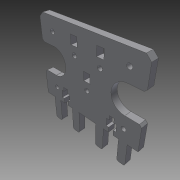
# Autodesk Inventor part: x_carryage_extruder_mount
Saved by Autodesk Inventor 2014 (Build 180170000, 170)
## iProperties
Created: 2014-03-26
Part Number: x_carryage_extruder_mount
Material: Generic
Document SubType Name: Modeling
Designer: buben
Density: 1 g/cm^3
Appearance: Default
Mass: 39.8284 g
Surface Area: 154.479 cm^2
Volume: 39.8284 cm^3
Author: buben
Autodesk Inventor part; units mm, degrees
ref_plane "YZ Plane" through (0, 0, 0) normal (1, 0, 0) x (0, 1, 0)
ref_plane "XZ Plane" through (0, 0, 0) normal (0, 1, 0) x (-1, 0, 0)
ref_plane "XY Plane" through (0, 0, 0) normal (0, 0, 1) x (1, 0, 0)
sketch "Sketch1" plane through (0, 0, 0) normal (0, 1, 0) x (-1, 0, 0)
  line L0 (0, 0) -> (-100, 0)
  line L1 (-100, 0) -> (-100, -24.25)
  line L2 (-100, -24.25) -> (-86, -24.25)
  arc A0 (-86, -50.25) -> (-86, -24.25) centre (-86, -37.25) ccw
  line L3 (-86, -50.25) -> (-100, -50.25)
  line L4 (-100, -50.25) -> (-100, -74.5)
  line L5 (-100, -74.5) -> (0, -74.5)
  line L6 (0, -74.5) -> (0, -50.25)
  line L7 (0, -50.25) -> (-14, -50.25)
  arc A1 (-14, -24.25) -> (-14, -50.25) centre (-14, -37.25) ccw
  line L8 (-14, -24.25) -> (0, -24.25)
  line L9 (0, -24.25) -> (0, 0)
  circle A2 centre (-14, -62.25) radius 2.25
  circle A3 centre (-14, -12.25) radius 2.25
  circle A4 centre (-86, -62.25) radius 2.25
  circle A5 centre (-86, -12.25) radius 2.25
  dimension "d0" = 13
  dimension "d1" = 50
  dimension "d2" = 4.5
  dimension "d3" = 25
  dimension "d5" = 12.25
  dimension "d6" = 100
  dimension "d10" = 14
  constraints: 20 end point, 7 collinear, 6 centre point, 4 parallel, 4 perpendicular, 4 point on circle, 4 tangent, 4 vertical alignment, 3 equal radius, 2 horizontal alignment, 1 horizontal
  measures "d0" radius of A1
  measures "d1" distance of A3.centre A2.centre
  measures "d2" diameter of A2
  measures "d3" distance of A1.centre A2.centre
  measures "d5" distance from line of L5 A2.centre
  measures "d6" distance of L0.start L0.end
  measures "d10" distance from line of L9 A3.centre
extrude "Extrusion1" add sketch "Sketch1" along normal blind 6.5
sketch "Sketch3" plane through (0, 6.5, 0) normal (0, 1, 0) x (1, 0, 0)
  line L0 (100, 74.5) -> (0, 74.5) projected
  line L1 (22.75, 74.5) -> (27.25, 74.5)
  line L2 (27.25, 58.2) -> (22.75, 58.2)
  line L3 (29.75, 69.5) -> (29.75, 62.2)
  line L4 (20.25, 62.2) -> (20.25, 69.5)
  line L5 (27.25, 74.5) -> (27.25, 69.5)
  line L6 (27.25, 62.2) -> (27.25, 58.2)
  line L7 (22.75, 58.2) -> (22.75, 62.2)
  line L8 (22.75, 69.5) -> (22.75, 74.5)
  line L9 (20.25, 69.5) -> (22.75, 69.5)
  line L10 (27.25, 69.5) -> (29.75, 69.5)
  line L11 (29.75, 62.2) -> (27.25, 62.2)
  line L12 (22.75, 62.2) -> (20.25, 62.2)
  line L13 (72.75, 74.5) -> (77.25, 74.5)
  line L14 (77.25, 58.2) -> (72.75, 58.2)
  line L15 (79.75, 69.5) -> (79.75, 62.2)
  line L16 (70.25, 62.2) -> (70.25, 69.5)
  line L17 (77.25, 74.5) -> (77.25, 69.5)
  line L18 (77.25, 62.2) -> (77.25, 58.2)
  line L19 (72.75, 58.2) -> (72.75, 62.2)
  line L20 (72.75, 69.5) -> (72.75, 74.5)
  line L21 (70.25, 69.5) -> (72.75, 69.5)
  line L22 (77.25, 69.5) -> (79.75, 69.5)
  line L23 (79.75, 62.2) -> (77.25, 62.2)
  line L24 (72.75, 62.2) -> (70.25, 62.2)
  line L25 (29.75, 65.85) -> (70.25, 65.85) construction
  point P0 (25, 58.2)
  point P1 (75, 58.2)
  point P2 (50, 65.85)
  point P3 (50, 74.5)
  dimension "d15" = 4.5
  dimension "d16" = 2.5
  dimension "d17" = 4
  dimension "d18" = 5
  dimension "d19" = 7.3
  dimension "d20" = 4.5
  dimension "d21" = 2.5
  dimension "d22" = 4
  dimension "d23" = 5
  dimension "d24" = 7.3
  dimension "d25" = 50
  constraints: 50 end point, 20 parallel, 12 collinear, 8 perpendicular, 6 horizontal, 6 midpoint, 1 vertical alignment
  measures "d15" distance of L2.start L2.end
  measures "d16" distance of L7.end L4.start
  measures "d17" distance of L2.end L7.end
  measures "d18" distance of L8.start L1.start
  measures "d19" distance of L4.start L4.end
  measures "d20" distance of L18.end L19.start
  measures "d21" distance of L24.start L24.end
  measures "d22" distance of L19.start L24.start
  measures "d23" distance of L20.start L20.end
  measures "d24" distance of L24.end L21.start
  measures "d25" distance of point (75, 58.2) point (25, 58.2)
extrude "Extrusion2" cut sketch "Sketch3" against normal through all
sketch "Sketch4" plane through (0, 6.5, 0) normal (0, 1, 0) x (1, 0, 0)
  line L0 (22.75, 74.5) -> (0, 74.5) projected
  line L1 (100, 74.5) -> (77.25, 74.5) projected
  line L2 (77.25, 58.2) -> (72.75, 58.2) projected
  line L3 (72.75, 74.5) -> (27.25, 74.5) projected
  line L4 (27.25, 58.2) -> (22.75, 58.2) projected
  line L5 (9.5, 74.5) -> (17.5, 74.5)
  line L6 (17.5, 74.5) -> (17.5, 95.7)
  line L7 (15.5, 97.7) -> (11.5, 97.7)
  line L8 (9.5, 95.7) -> (9.5, 74.5)
  line L9 (32.5, 74.5) -> (40.5, 74.5)
  line L10 (40.5, 74.5) -> (40.5, 95.7)
  line L11 (38.5, 97.7) -> (34.5, 97.7)
  line L12 (32.5, 95.7) -> (32.5, 74.5)
  line L13 (59.5, 74.5) -> (67.5, 74.5)
  line L14 (67.5, 74.5) -> (67.5, 95.7)
  line L15 (65.5, 97.7) -> (61.5, 97.7)
  line L16 (59.5, 95.7) -> (59.5, 74.5)
  line L17 (82.5, 74.5) -> (90.5, 74.5)
  line L18 (90.5, 74.5) -> (90.5, 95.7)
  line L19 (88.5, 97.7) -> (84.5, 97.7)
  line L20 (82.5, 95.7) -> (82.5, 74.5)
  arc A0 (11.5, 97.7) -> (9.5, 95.7) centre (11.5, 95.7) ccw
  arc A1 (17.5, 95.7) -> (15.5, 97.7) centre (15.5, 95.7) ccw
  arc A2 (34.5, 97.7) -> (32.5, 95.7) centre (34.5, 95.7) ccw
  arc A3 (40.5, 95.7) -> (38.5, 97.7) centre (38.5, 95.7) ccw
  arc A4 (61.5, 97.7) -> (59.5, 95.7) centre (61.5, 95.7) ccw
  arc A5 (67.5, 95.7) -> (65.5, 97.7) centre (65.5, 95.7) ccw
  arc A6 (84.5, 97.7) -> (82.5, 95.7) centre (84.5, 95.7) ccw
  arc A7 (90.5, 95.7) -> (88.5, 97.7) centre (88.5, 95.7) ccw
  point P0 (25, 58.2)
  point P1 (75, 58.2)
  dimension "d28" = 2
  dimension "d29" = 23.2
  dimension "d30" = 8
  dimension "d31" = 8
  dimension "d32" = 8
  dimension "d33" = 8
  dimension "d34" = 15
  dimension "d35" = 15
  dimension "d36" = 7.5
  dimension "d37" = 7.5
  constraints: 32 end point, 16 point on circle, 16 tangent, 8 centre point, 8 parallel, 7 equal radius, 4 horizontal, 4 perpendicular, 4 point on line, 3 collinear, 2 midpoint
  measures "d28" radius of A0
  measures "d29" distance between parallel lines of L0 L7
  measures "d30" distance between parallel lines of L6 L8
  measures "d31" distance between parallel lines of L10 L12
  measures "d32" distance between parallel lines of L14 L16
  measures "d33" distance between parallel lines of L18 L20
  measures "d34" distance between parallel lines of L12 L6
  measures "d35" distance between parallel lines of L20 L14
  measures "d36" distance from line of point (25, 58.2) L6
  measures "d37" distance from line of L14 point (75, 58.2)
extrude "Extrusion3" add sketch "Sketch4" against normal blind 6.5
chamfer "Chamfer1" distance 4 angle 45 2 edges at (100, 3.25, 0) (0, 3.25, 0)
chamfer "Chamfer2" distance 2 angle 45 4 edges at (100, 3.25, -24.25) (100, 3.25, -50.25) (0, 3.25, -50.25) (0, 3.25, -24.25)
sketch "Sketch5" plane through (0, 6.5, 0) normal (0, 1, 0) x (1, 0, 0)
  line L0 (4, 0) -> (96, 0) projected
  line L1 (34.25, 16) -> (40.75, 16)
  line L2 (40.75, 16) -> (40.75, 8)
  line L3 (40.75, 8) -> (34.25, 8)
  line L4 (34.25, 8) -> (34.25, 16)
  line L5 (59.25, 16) -> (65.75, 16)
  line L6 (65.75, 16) -> (65.75, 8)
  line L7 (65.75, 8) -> (59.25, 8)
  line L8 (59.25, 8) -> (59.25, 16)
  circle A0 centre (37.5, 23.5) radius 2.25
  circle A1 centre (62.5, 23.5) radius 2.25
  line L9 (37.5, 23.5) -> (62.5, 23.5) construction
  point P0 (0, 0)
  point P1 (37.5, 16)
  point P2 (62.5, 16)
  point P3 (50, 23.5)
  point P4 (50, 0)
  dimension "d46" = 4.5
  dimension "d47" = 6.5
  dimension "d48" = 8
  dimension "d49" = 25
  dimension "d50" = 8
  dimension "d51" = 7.5
  constraints: 18 end point, 4 midpoint, 4 parallel, 3 collinear, 3 perpendicular, 3 vertical alignment, 2 centre point, 2 horizontal, 1 equal radius, 1 horizontal alignment
  measures "d46" diameter of A0
  measures "d47" distance of L1.start L1.end
  measures "d48" distance of L3.end L1.start
  measures "d49" distance of L9.end L9.start
  measures "d50" distance between parallel lines of L0 L3
  measures "d51" distance from line of L1 L9.start
extrude "Extrusion4" cut sketch "Sketch5" against normal through all
sketch "Sketch6" plane through (0, 6.5, 0) normal (0, 1, 0) x (1, 0, 0)
  line L0 (59.5, 74.5) -> (40.5, 74.5) projected
  line L1 (46.75, 40.5) -> (53.25, 40.5)
  line L2 (53.25, 40.5) -> (53.25, 32.5)
  line L3 (53.25, 32.5) -> (46.75, 32.5)
  line L4 (46.75, 32.5) -> (46.75, 40.5)
  circle A0 centre (50, 48) radius 2.25
  point P0 (0, 0)
  point P1 (50, 74.5)
  point P2 (50, 40.5)
  dimension "d54" = 6.5
  dimension "d55" = 8
  dimension "d56" = 4.5
  dimension "d57" = 7.5
  dimension "d58" = 34
  constraints: 8 end point, 2 midpoint, 2 parallel, 2 vertical alignment, 1 centre point, 1 horizontal, 1 perpendicular
  measures "d54" distance of L2.end L3.end
  measures "d55" distance of L3.end L1.start
  measures "d56" diameter of A0
  measures "d57" distance from line of A0.centre L1
  measures "d58" distance between parallel lines of L0 L1
extrude "Extrusion5" cut sketch "Sketch6" against normal through all
equation "\"d3\" = 0.5 * d1"
equation "\"d31\" = d30"
equation "\"d32\" = d31"
equation "\"d33\" = d32"
equation "\"d36\" = 0.5 * d34"
equation "\"d37\" = 0.5 * d35"
body "Solid1"
